Autodesk Inventor part; units mm, degrees
(part 2 of 2)
  line L239 (17.6502, -12.8499) -> (18.2403, -9.7183)
  line L240 (18.2403, -9.7183) -> (21.2697, -9.7183)
  line L241 (21.2697, -9.7183) -> (21.2697, -10.4338)
  line L242 (21.2697, -10.4338) -> (18.8397, -10.4338)
  line L243 (18.8397, -10.4338) -> (18.5098, -12.0693)
  spline S304 degree 2 poles (18.5098, -12.0693) (19.058, -11.6883) (19.6621, -11.6883) knots 0 0 0 1 1 1
  spline S305 degree 2 poles (19.6621, -11.6883) (20.4612, -11.6883) (21.5578, -12.7941) (21.5578, -13.663) knots 0 0 0 1 2 2 2
  spline S306 degree 2 poles (21.5578, -13.663) (21.5578, -14.4947) (21.0746, -15.0987) knots 0 0 0 1 1 1
  spline S307 degree 2 poles (21.0746, -15.0987) (20.4891, -15.8375) (19.4762, -15.8375) knots 0 0 0 1 1 1
  spline S308 degree 2 poles (19.4762, -15.8375) (18.6445, -15.8375) (17.5898, -14.9082) (17.5155, -14.1369) knots 0 0 0 1 2 2 2
  line L244 (-1.8319, -25.3286) -> (-1.8319, -19.2326)
  line L245 (-1.8319, -19.2326) -> (-1.0049, -19.2326)
  line L246 (-1.0049, -19.2326) -> (2.2011, -24.0183)
  line L247 (2.2011, -24.0183) -> (2.2011, -19.2326)
  line L248 (2.2011, -19.2326) -> (2.9724, -19.2326)
  line L249 (2.9724, -19.2326) -> (2.9724, -25.3286)
  line L250 (2.9724, -25.3286) -> (2.1454, -25.3286)
  line L251 (2.1454, -25.3286) -> (-1.0606, -20.5428)
  line L252 (-1.0606, -20.5428) -> (-1.0606, -25.3286)
  line L253 (-1.0606, -25.3286) -> (-1.8319, -25.3286)
  point P0 (0, 0)
  constraints: 2 other
emboss "Emboss1" sketch "Sketch2" operation cut depth 1.5 direction (0, 0, -1)
sketch "Sketch3" plane through (0, 0, 0) normal (0, 0, -1) x (-1, 0, 0)
  line L0 (-20.876, 15.9739) -> (21.3831, 15.9739) construction
  line L1 (21.3831, 15.9739) -> (21.3831, -18.8475) construction
  line L2 (21.3831, -18.8475) -> (-20.876, -18.8475) construction
  line L3 (-20.876, -18.8475) -> (-20.876, 15.9739) construction
  point P0 (0, 0)
  constraints: 2 other
body "Solid1"
